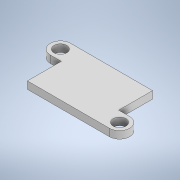
# Autodesk Inventor part: USB Mount
Saved by Autodesk Inventor 2020 (Build 240168000, 168)
## iProperties
Created: 2020-02-13
Part Number: USB Mount
Material: Generic
Document SubType Name: Modeling
Designer: pp445
Density: 1 g/cm^3
Appearance: Default
Author: pp445
Autodesk Inventor part; units mm, degrees
ref_plane "YZ Plane" through (0, 0, 0) normal (1, 0, 0) x (0, 1, 0)
ref_plane "XZ Plane" through (0, 0, 0) normal (0, 1, 0) x (-1, 0, 0)
ref_plane "XY Plane" through (0, 0, 0) normal (0, 0, 1) x (1, 0, 0)
sketch "Sketch1" plane through (0, 0, 0) normal (0, 1, 0) x (-1, 0, 0)
  line L0 (0, 0) -> (17.272, 0)
  line L1 (17.272, 0) -> (17.272, -12.7)
  line L2 (17.272, -12.7) -> (0, -12.7)
  line L3 (0, -12.7) -> (0, 0)
  circle A0 centre (21.272, -10.95) radius 1.75
  circle A1 centre (-4, -1.75) radius 1.75
  line L4 (17.272, -6.35) -> (0, -6.35) construction
  circle A2 centre (21.272, -10.95) radius 2.75
  line L5 (18.272, -13.7) -> (18.272, 1)
  line L6 (18.272, 1) -> (-1, 1)
  line L7 (-1, 1) -> (-1, -13.7)
  line L8 (-1, -13.7) -> (18.272, -13.7)
  line L9 (18.272, -13.7) -> (21.272, -13.7)
  line L10 (21.272, -8.2) -> (18.272, -8.2)
  circle A3 centre (-4, -1.75) radius 2.75
  line L11 (-1, 1) -> (-4, 1)
  line L12 (-4, -4.5) -> (-1, -4.5)
  dimension "d0" = 17.272
  dimension "d1" = 12.7
  dimension "d2" = 3.5
  dimension "d3" = 3.5
  dimension "d4" = 4
  dimension "d5" = 4
  dimension "d6" = 5.5
  dimension "d7" = 5.5
  constraints: 26 end point, 7 tangent, 4 centre point, 4 parallel, 4 perpendicular, 4 point on circle, 2 coincident, 2 midpoint, 2 point on line, 1 horizontal, 3 other
  measures "d0" distance of L0.start L0.end
  measures "d1" distance of L0.end L1.end
  measures "d2" diameter of A1
  measures "d3" diameter of A0
  measures "d4" distance from line of L3 A1.centre
  measures "d5" distance from line of L1 A0.centre
  measures "d6" diameter of A2
  measures "d7" diameter of A3
extrude "Extrusion1" add sketch "Sketch1" along normal blind 2 contours L0 L1 L2 L3 | A2 | A2 L9 L5 L10 | L5 L8 L7 L6 | L7 L12 A3 L11 | A3
equation "\"d3\" = d2"
equation "\"d5\" = d4"
equation "\"d7\" = d6"
body "Solid1"
